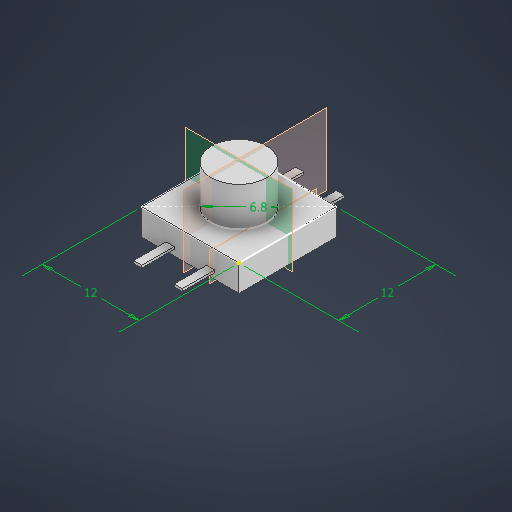
# Autodesk Inventor part: Button
Saved by Autodesk Inventor 2025.2 (Build 292293000, 293)
## iProperties
Created: 2024-11-19
Part Number: Button
Material: Generic
Document SubType Name: Modeling
Designer: JL
Density: 1 g/cm^3
Appearance: Default
Author: JL
Autodesk Inventor part; units mm, degrees
ref_plane "YZ Plane" through (0, 0, 0) normal (1, 0, 0) x (0, 1, 0)
ref_plane "XZ Plane" through (0, 0, 0) normal (0, 1, 0) x (-1, 0, 0)
ref_plane "XY Plane" through (0, 0, 0) normal (0, 0, 1) x (1, 0, 0)
sketch "Sketch1" plane through (0, 0, 0) normal (0, 1, 0) x (-1, 0, 0)
  line L0 (12, -12) -> (0, -12)
  line L1 (0, -12) -> (0, 0)
  line L2 (0, 0) -> (12, 0)
  line L3 (12, 0) -> (12, -12)
  circle A0 centre (6, -6) radius 3.4
  line L4 (12, 0) -> (0, -12) construction
  point P0 (6, -6)
  dimension "d0" = 12
  dimension "d1" = 12
  dimension "d4" = 6.8
  constraints: 10 end point, 2 coincident, 2 parallel, 1 centre point, 1 horizontal, 1 midpoint, 1 perpendicular
  measures "d0" distance of L1.end L2.end
  measures "d1" distance of L0.end L1.end
  measures "d4" diameter of A0
extrude "Extrusion1" add sketch "Sketch1" against normal blind 3.25 contours L0 L1 L2 L3 | A0
extrude "Extrusion2" add sketch "Sketch1" along normal blind 4.8 contours A0
ref_plane "Work Plane1" through (-3, 0, 0) normal (1, 0, 0) x (0, 0, -1)
sketch "Sketch2" plane through (-3, 0, 0) normal (1, 0, 0) x (0, 0, -1)
  line L0 (12, -3.25) -> (0, -3.25) projected
  line L1 (12, -2.55) -> (16, -2.55)
  line L2 (16, -2.55) -> (16, -2.25)
  line L3 (16, -2.25) -> (12, -2.25)
  line L4 (12, -2.25) -> (12, -2.55)
  line L5 (12, 0) -> (12, -3.25) projected
  point P0 (0, 0)
  dimension "d8" = 4
  dimension "d9" = 0.3
  dimension "d10" = 0.7
  constraints: 8 end point, 2 parallel, 1 collinear, 1 horizontal, 1 perpendicular
  measures "d8" distance of L3.end L2.end
  measures "d9" distance of L2.end L1.end
  measures "d10" distance of L0.start L1.start
extrude "Extrusion3" add sketch "Sketch2" against normal blind 1
ref_plane "Work Plane2" through (-6, 0, 0) normal (1, 0, 0) x (0, 0, -1)
ref_plane "Work Plane3" through (0, 0, -6) normal (0, 0, -1) x (-1, 0, 0)
mirror "Mirror1" about plane through (-6, 0, 0) normal (1, 0, 0) of "Extrusion3"
mirror "Mirror2" about plane through (0, 0, -6) normal (0, 0, -1) of "Extrusion3", "Mirror1"
body "Solid1"
